Autodesk Fusion 360 part; units mm, degrees
note: some values were not read from the file. Set by a fixed rule: which face or edge a step refers to.
(part 2 of 2)
  spline S350 degree 3 poles (3.3037, -76.5729) (2.2719, -76.176) (1.5046, -77.2079) (2.1131, -78.1604) knots 0 0 0 0 1 1 1 1
  spline S351 degree 3 poles (2.1131, -78.1604) (2.4042, -78.6367) (4.9971, -78.769) (6.2142, -78.3456) knots 0 0 0 0 1 1 1 1
  spline S352 degree 3 poles (2.3248, -77.9488) (2.166, -77.79) (2.1131, -77.4725) (2.2189, -77.2344) knots 0 0 0 0 1 1 1 1
  spline S353 degree 3 poles (2.2189, -77.2344) (2.3512, -76.8904) (2.5894, -76.8375) (3.4889, -76.9698) knots 0 0 0 0 1 1 1 1
  spline S354 degree 3 poles (3.4889, -76.9698) (4.2298, -77.0756) (5.0235, -76.9963) (5.7908, -76.7052) knots 0 0 0 0 1 1 1 1
  spline S355 degree 3 poles (5.7908, -76.7052) (6.7962, -76.3613) (7.0344, -76.3613) (7.3254, -76.6523) knots 0 0 0 0 1 1 1 1
  spline S356 degree 3 poles (7.3254, -76.6523) (7.6164, -76.9433) (7.6164, -77.0756) (7.2196, -77.4196) knots 0 0 0 0 1 1 1 1
  spline S357 degree 3 poles (7.2196, -77.4196) (6.2142, -78.3456) (3.0392, -78.6631) (2.3248, -77.9488) knots 0 0 0 0 1 1 1 1
  spline S358 degree 3 poles (-4.3956, -78.425) (-3.0463, -78.1869) (-2.7552, -76.7052) (-3.9723, -76.3877) knots 0 0 0 0 1 1 1 1
  spline S359 degree 3 poles (-3.9723, -76.3877) (-4.475, -76.2554) (-4.475, -76.229) (-3.8929, -75.7263) knots 0 0 0 0 1 1 1 1
  line L74 (-3.8929, -75.7263) -> (-3.3108, -75.1971)
  line L75 (-3.3108, -75.1971) -> (-3.9723, -75.6204)
  spline S360 degree 3 poles (-3.9723, -75.6204) (-4.9248, -76.229) (-6.0096, -76.1496) (-6.7504, -75.3823) knots 0 0 0 0 1 1 1 1
  spline S361 degree 3 poles (-6.7504, -75.3823) (-7.5706, -74.5885) (-7.5971, -73.7154) (-6.8563, -72.71) knots 0 0 0 0 1 1 1 1
  line L76 (-6.8563, -72.71) -> (-6.3006, -71.9427)
  line L77 (-6.3006, -71.9427) -> (-6.9886, -72.6835)
  spline S362 degree 3 poles (-6.9886, -72.6835) (-7.359, -73.0804) (-7.6765, -73.7154) (-7.6765, -74.0858) knots 0 0 0 0 1 1 1 1
  spline S363 degree 3 poles (-7.6765, -74.0858) (-7.6765, -74.9854) (-6.3271, -76.3083) (-5.3746, -76.3348) knots 0 0 0 0 1 1 1 1
  spline S364 degree 3 poles (-5.3746, -76.3348) (-4.8983, -76.3613) (-4.7925, -76.4142) (-5.11, -76.4935) knots 0 0 0 0 1 1 1 1
  spline S365 degree 3 poles (-5.11, -76.4935) (-5.3746, -76.5729) (-6.1948, -76.4142) (-6.9356, -76.176) knots 0 0 0 0 1 1 1 1
  spline S366 degree 3 poles (-6.9356, -76.176) (-7.9411, -75.8585) (-8.3379, -75.8321) (-8.629, -76.0702) knots 0 0 0 0 1 1 1 1
  spline S367 degree 3 poles (-8.629, -76.0702) (-10.1106, -77.2873) (-7.1738, -78.9277) (-4.3956, -78.425) knots 0 0 0 0 1 1 1 1
  spline S368 degree 3 poles (-8.0204, -77.6313) (-9.4492, -76.9433) (-8.6819, -75.885) (-7.2002, -76.4935) knots 0 0 0 0 1 1 1 1
  spline S369 degree 3 poles (-7.2002, -76.4935) (-6.6711, -76.7052) (-5.7186, -76.8375) (-4.9248, -76.7846) knots 0 0 0 0 1 1 1 1
  spline S370 degree 3 poles (-4.9248, -76.7846) (-3.7871, -76.7052) (-3.5754, -76.7846) (-3.4961, -77.2079) knots 0 0 0 0 1 1 1 1
  spline S371 degree 3 poles (-3.4961, -77.2079) (-3.4431, -77.4725) (-3.549, -77.8165) (-3.7606, -77.9488) knots 0 0 0 0 1 1 1 1
  spline S372 degree 3 poles (-3.7606, -77.9488) (-4.2104, -78.2663) (-7.0944, -78.0546) (-8.0204, -77.6313) knots 0 0 0 0 1 1 1 1
  spline S373 degree 3 poles (-14.5027, -76.52) (-14.3175, -76.176) (-14.1588, -75.0119) (-14.1323, -73.7948) knots 0 0 0 0 1 1 1 1
  spline S374 degree 3 poles (-14.1323, -73.7948) (-14.1323, -72.419) (-13.9471, -71.3342) (-13.6825, -70.6992) knots 0 0 0 0 1 1 1 1
  spline S375 degree 3 poles (-13.6825, -70.6992) (-13.4444, -70.1435) (-13.2327, -69.6144) (-13.2327, -69.4821) knots 0 0 0 0 1 1 1 1
  spline S376 degree 3 poles (-13.2327, -69.4821) (-13.2327, -69.3498) (-13.0475, -69.0852) (-12.8358, -68.9) knots 0 0 0 0 1 1 1 1
  spline S377 degree 3 poles (-12.8358, -68.9) (-12.5448, -68.6619) (-12.2273, -68.6883) (-11.3013, -69.0323) knots 0 0 0 0 1 1 1 1
  spline S378 degree 3 poles (-11.3013, -69.0323) (-10.0842, -69.4821) (-5.745, -69.7202) (-4.475, -69.3763) knots 0 0 0 0 1 1 1 1
  spline S379 degree 3 poles (-4.475, -69.3763) (-3.9194, -69.2175) (-3.7342, -69.2969) (-3.4431, -69.826) knots 0 0 0 0 1 1 1 1
  spline S380 degree 3 poles (-3.4431, -69.826) (-3.0198, -70.5933) (-1.6704, -71.2813) (-0.5327, -71.2813) knots 0 0 0 0 1 1 1 1
  spline S381 degree 3 poles (-0.5327, -71.2813) (0.6314, -71.2813) (2.0602, -70.5404) (2.4835, -69.7467) knots 0 0 0 0 1 1 1 1
  spline S382 degree 3 poles (2.4835, -69.7467) (2.8275, -69.0588) (2.8275, -69.0588) (1.0019, -68.4502) knots 0 0 0 0 1 1 1 1
  spline S383 degree 3 poles (1.0019, -68.4502) (-0.2681, -68.0269) (-0.9561, -67.8946) (-1.1677, -68.0798) knots 0 0 0 0 1 1 1 1
  spline S384 degree 3 poles (-1.1677, -68.0798) (-1.3529, -68.2385) (-2.3319, -68.556) (-3.3373, -68.7942) knots 0 0 0 0 1 1 1 1
  spline S385 degree 3 poles (-3.3373, -68.7942) (-5.5069, -69.2969) (-9.555, -69.1646) (-11.3542, -68.5296) knots 0 0 0 0 1 1 1 1
  spline S386 degree 3 poles (-11.3542, -68.5296) (-12.9946, -67.921) (-13.1269, -67.974) (-13.4708, -69.244) knots 0 0 0 0 1 1 1 1
  spline S387 degree 3 poles (-13.4708, -69.244) (-13.6296, -69.879) (-13.9736, -70.6992) (-14.2646, -71.0431) knots 0 0 0 0 1 1 1 1
  spline S388 degree 3 poles (-14.2646, -71.0431) (-14.7144, -71.6252) (-14.7408, -71.8633) (-14.5027, -73.0804) knots 0 0 0 0 1 1 1 1
  spline S389 degree 3 poles (-14.5027, -73.0804) (-14.2911, -74.1652) (-14.3175, -74.6944) (-14.635, -75.6998) knots 0 0 0 0 1 1 1 1
  spline S390 degree 3 poles (-14.635, -75.6998) (-15.1113, -77.1021) (-15.0319, -77.4725) (-14.5027, -76.52) knots 0 0 0 0 1 1 1 1
  line L78 (-2.8611, -70.0642) -> (-3.4696, -69.3498)
  line L79 (-3.4696, -69.3498) -> (-2.0938, -68.9)
  spline S391 degree 3 poles (-2.0938, -68.9) (-0.5063, -68.3444) (-0.4004, -68.3444) (0.7373, -69.0323) knots 0 0 0 0 1 1 1 1
  spline S392 degree 3 poles (0.7373, -69.0323) (1.7692, -69.6408) (1.7162, -69.9319) (0.4992, -70.5669) knots 0 0 0 0 1 1 1 1
  spline S393 degree 3 poles (0.4992, -70.5669) (-0.6915, -71.2019) (-2.0673, -70.9902) (-2.8611, -70.0642) knots 0 0 0 0 1 1 1 1
  spline S394 degree 3 poles (2.0337, -69.5615) (2.1131, -69.3233) (2.2454, -69.191) (2.2983, -69.2704) knots 0 0 0 0 1 1 1 1
  spline S395 degree 3 poles (2.2983, -69.2704) (2.3777, -69.3498) (2.3512, -69.5085) (2.2454, -69.6673) knots 0 0 0 0 1 1 1 1
  spline S396 degree 3 poles (2.2454, -69.6673) (2.0073, -70.0906) (1.8485, -70.0113) (2.0337, -69.5615) knots 0 0 0 0 1 1 1 1
  spline S397 degree 3 poles (-0.2681, -70.514) (-0.2681, -70.3817) (0.0229, -70.1965) (0.3933, -70.1171) knots 0 0 0 0 1 1 1 1
  spline S398 degree 3 poles (0.3933, -70.1171) (0.7637, -70.0113) (1.0548, -69.826) (1.0548, -69.6938) knots 0 0 0 0 1 1 1 1
  spline S399 degree 3 poles (1.0548, -69.6938) (1.0548, -69.5615) (0.7373, -69.5615) (0.261, -69.7202) knots 0 0 0 0 1 1 1 1
  spline S400 degree 3 poles (0.261, -69.7202) (-0.1888, -69.879) (-0.5327, -70.17) (-0.5327, -70.3817) knots 0 0 0 0 1 1 1 1
  spline S401 degree 3 poles (-0.5327, -70.3817) (-0.5327, -70.5933) (-0.4798, -70.7521) (-0.4004, -70.7521) knots 0 0 0 0 1 1 1 1
  spline S402 degree 3 poles (-0.4004, -70.7521) (-0.3211, -70.7521) (-0.2681, -70.6463) (-0.2681, -70.514) knots 0 0 0 0 1 1 1 1
  spline S403 degree 3 poles (4.0446, -76.0438) (3.5683, -75.9379) (3.0127, -75.7527) (2.8275, -75.6204) knots 0 0 0 0 1 1 1 1
  spline S404 degree 3 poles (2.8275, -75.6204) (2.6423, -75.4881) (2.7217, -75.594) (2.9862, -75.8585) knots 0 0 0 0 1 1 1 1
  spline S405 degree 3 poles (2.9862, -75.8585) (3.2773, -76.0967) (3.8064, -76.3083) (4.2033, -76.2819) knots 0 0 0 0 1 1 1 1
  spline S406 degree 3 poles (4.2033, -76.2819) (4.8383, -76.2554) (4.8119, -76.229) (4.0446, -76.0438) knots 0 0 0 0 1 1 1 1
  spline S407 degree 3 poles (5.8967, -75.5675) (6.1612, -75.3029) (6.3464, -74.8531) (6.32, -74.5621) knots 0 0 0 0 1 1 1 1
  spline S408 degree 3 poles (6.32, -74.5621) (6.32, -74.1917) (6.2671, -74.1652) (6.1612, -74.4563) knots 0 0 0 0 1 1 1 1
  spline S409 degree 3 poles (6.1612, -74.4563) (6.0819, -74.6679) (5.7644, -75.1177) (5.4733, -75.4617) knots 0 0 0 0 1 1 1 1
  spline S410 degree 3 poles (5.4733, -75.4617) (5.1823, -75.7792) (5.05, -76.0438) (5.2087, -76.0438) knots 0 0 0 0 1 1 1 1
  spline S411 degree 3 poles (5.2087, -76.0438) (5.341, -76.0438) (5.6585, -75.8321) (5.8967, -75.5675) knots 0 0 0 0 1 1 1 1
  spline S412 degree 3 poles (-3.9458, -74.6944) (-3.2315, -73.98) (-3.3638, -72.8688) (-4.2633, -72.366) knots 0 0 0 0 1 1 1 1
  spline S413 degree 3 poles (-4.2633, -72.366) (-4.8983, -72.0221) (-5.0306, -72.0221) (-5.6656, -72.419) knots 0 0 0 0 1 1 1 1
  spline S414 degree 3 poles (-5.6656, -72.419) (-6.38, -72.8952) (-6.6446, -74.2446) (-6.089, -74.5885) knots 0 0 0 0 1 1 1 1
  spline S415 degree 3 poles (-6.089, -74.5885) (-5.9567, -74.6679) (-5.8244, -74.615) (-5.8244, -74.4827) knots 0 0 0 0 1 1 1 1
  spline S416 degree 3 poles (-5.8244, -74.4827) (-5.8244, -74.324) (-5.6392, -74.1917) (-5.4011, -74.1917) knots 0 0 0 0 1 1 1 1
  spline S417 degree 3 poles (-5.4011, -74.1917) (-5.11, -74.1917) (-5.0042, -74.3504) (-5.11, -74.7208) knots 0 0 0 0 1 1 1 1
  spline S418 degree 3 poles (-5.11, -74.7208) (-5.2952, -75.4352) (-4.6602, -75.4088) (-3.9458, -74.6944) knots 0 0 0 0 1 1 1 1
  spline S419 degree 3 poles (-5.3746, -73.2392) (-5.3481, -73.1069) (-5.0836, -72.9746) (-4.819, -72.9217) knots 0 0 0 0 1 1 1 1
  spline S420 degree 3 poles (-4.819, -72.9217) (-4.2898, -72.8423) (-3.84, -73.5038) (-4.1311, -73.9535) knots 0 0 0 0 1 1 1 1
  spline S421 degree 3 poles (-4.1311, -73.9535) (-4.3163, -74.271) (-5.454, -73.5831) (-5.3746, -73.2392) knots 0 0 0 0 1 1 1 1
  spline S422 degree 3 poles (3.8594, -74.7473) (3.78, -74.615) (3.8858, -74.3769) (4.071, -74.2181) knots 0 0 0 0 1 1 1 1
  spline S423 degree 3 poles (4.071, -74.2181) (4.3621, -73.9535) (4.5208, -74.0065) (4.706, -74.3769) knots 0 0 0 0 1 1 1 1
  spline S424 degree 3 poles (4.706, -74.3769) (4.9442, -74.8002) (4.9971, -74.7473) (5.1823, -74.0858) knots 0 0 0 0 1 1 1 1
  spline S425 degree 3 poles (5.1823, -74.0858) (5.4998, -72.7629) (4.4944, -71.784) (3.2508, -72.2338) knots 0 0 0 0 1 1 1 1
  spline S426 degree 3 poles (3.2508, -72.2338) (1.9544, -72.6835) (2.1396, -74.9854) (3.4889, -74.9854) knots 0 0 0 0 1 1 1 1
  spline S427 degree 3 poles (3.4889, -74.9854) (3.7535, -74.9854) (3.9387, -74.8796) (3.8594, -74.7473) knots 0 0 0 0 1 1 1 1
  spline S428 degree 3 poles (3.0921, -73.4508) (3.3302, -72.8158) (3.7535, -72.5777) (4.1504, -72.9217) knots 0 0 0 0 1 1 1 1
  spline S429 degree 3 poles (4.1504, -72.9217) (4.415, -73.1333) (4.3621, -73.2921) (3.8858, -73.6625) knots 0 0 0 0 1 1 1 1
  spline S430 degree 3 poles (3.8858, -73.6625) (3.2244, -74.2181) (2.8539, -74.1123) (3.0921, -73.4508) knots 0 0 0 0 1 1 1 1
  spline S431 degree 3 poles (6.32, -73.3715) (6.3464, -73.1333) (6.0819, -72.7365) (5.7379, -72.4454) knots 0 0 0 0 1 1 1 1
  spline S432 degree 3 poles (5.7379, -72.4454) (5.1558, -71.9427) (5.1558, -71.9427) (5.5792, -72.4719) knots 0 0 0 0 1 1 1 1
  spline S433 degree 3 poles (5.5792, -72.4719) (5.8173, -72.7629) (6.0819, -73.1863) (6.1612, -73.3979) knots 0 0 0 0 1 1 1 1
  spline S434 degree 3 poles (6.1612, -73.3979) (6.2935, -73.7419) (6.32, -73.7419) (6.32, -73.3715) knots 0 0 0 0 1 1 1 1
  spline S435 degree 3 poles (13.2256, -65.3017) (13.2256, -63.4231) (7.881, -61.5446) (4.3092, -62.1796) knots 0 0 0 0 1 1 1 1
  spline S436 degree 3 poles (4.3092, -62.1796) (3.145, -62.3913) (3.2773, -62.4177) (5.9496, -62.5765) knots 0 0 0 0 1 1 1 1
  spline S437 degree 3 poles (5.9496, -62.5765) (7.5371, -62.6823) (9.2833, -62.894) (9.8125, -63.0527) knots 0 0 0 0 1 1 1 1
  spline S438 degree 3 poles (9.8125, -63.0527) (11.1089, -63.4496) (12.4848, -64.4021) (12.8817, -65.1958) knots 0 0 0 0 1 1 1 1
  spline S439 degree 3 poles (12.8817, -65.1958) (13.1992, -65.8308) (13.2256, -65.8308) (13.2256, -65.3017) knots 0 0 0 0 1 1 1 1
  spline S440 degree 3 poles (-13.8148, -64.6667) (-13.0475, -63.4231) (-10.0577, -62.55) (-6.5388, -62.55) knots 0 0 0 0 1 1 1 1
  spline S441 degree 3 poles (-6.5388, -62.55) (-4.819, -62.5235) (-4.475, -62.4706) (-4.8719, -62.2325) knots 0 0 0 0 1 1 1 1
  spline S442 degree 3 poles (-4.8719, -62.2325) (-5.5333, -61.8621) (-9.1846, -62.1267) (-11.0896, -62.7088) knots 0 0 0 0 1 1 1 1
  spline S443 degree 3 poles (-11.0896, -62.7088) (-12.3861, -63.0792) (-14.6086, -64.6931) (-14.2911, -65.0371) knots 0 0 0 0 1 1 1 1
  spline S444 degree 3 poles (-14.2911, -65.0371) (-14.2117, -65.1165) (-14, -64.9313) (-13.8148, -64.6667) knots 0 0 0 0 1 1 1 1
  spline S445 degree 3 poles (0.2081, -63.529) (0.7637, -63.2115) (0.6844, -63.185) (-0.5327, -63.185) knots 0 0 0 0 1 1 1 1
  spline S446 degree 3 poles (-0.5327, -63.185) (-1.7498, -63.185) (-1.8292, -63.2115) (-1.2736, -63.529) knots 0 0 0 0 1 1 1 1
  spline S447 degree 3 poles (-1.2736, -63.529) (-0.9296, -63.7142) (-0.6121, -63.8465) (-0.5327, -63.8465) knots 0 0 0 0 1 1 1 1
  spline S448 degree 3 poles (-0.5327, -63.8465) (-0.4533, -63.8465) (-0.1358, -63.7142) (0.2081, -63.529) knots 0 0 0 0 1 1 1 1
  spline S449 degree 3 poles (2.6158, -62.3648) (1.3458, -60.8567) (-2.7023, -60.8831) (-3.9988, -62.4442) knots 0 0 0 0 1 1 1 1
  spline S450 degree 3 poles (-3.9988, -62.4442) (-4.2633, -62.7617) (-3.7606, -62.8146) (-0.665, -62.8146) knots 0 0 0 0 1 1 1 1
  spline S451 degree 3 poles (-0.665, -62.8146) (2.6952, -62.8146) (2.9333, -62.7881) (2.6158, -62.3648) knots 0 0 0 0 1 1 1 1
  spline S452 degree 3 poles (-0.6121, -61.8356) (-0.4269, -61.7827) (-0.1094, -61.7827) (0.0494, -61.8356) knots 0 0 0 0 1 1 1 1
  spline S453 degree 3 poles (0.0494, -61.8356) (0.2346, -61.915) (0.1023, -61.9679) (-0.2681, -61.9679) knots 0 0 0 0 1 1 1 1
  spline S454 degree 3 poles (-0.2681, -61.9679) (-0.6386, -61.9679) (-0.7708, -61.915) (-0.6121, -61.8356) knots 0 0 0 0 1 1 1 1
  spline S455 degree 3 poles (0.896, -33.4723) (1.0812, -33.1813) (-0.1358, -32.9431) (-0.5327, -33.1813) knots 0 0 0 0 1 1 1 1
  spline S456 degree 3 poles (-0.5327, -33.1813) (-0.7444, -33.3135) (-0.6915, -33.4194) (-0.4004, -33.5517) knots 0 0 0 0 1 1 1 1
  spline S457 degree 3 poles (-0.4004, -33.5517) (0.2081, -33.7898) (0.7373, -33.7633) (0.896, -33.4723) knots 0 0 0 0 1 1 1 1
  spline S458 degree 3 poles (3.0656, -30.7206) (3.145, -30.509) (3.1714, -29.4242) (3.1185, -28.26) knots 0 0 0 0 1 1 1 1
  line L80 (3.1185, -28.26) -> (3.0392, -26.1698)
  line L81 (3.0392, -26.1698) -> (0.261, -26.1698)
  line L82 (0.261, -26.1698) -> (-2.5171, -26.1698)
  line L83 (-2.5171, -26.1698) -> (-2.5171, -28.551)
  line L84 (-2.5171, -28.551) -> (-2.5171, -30.9323)
  line L85 (-2.5171, -30.9323) -> (0.2081, -31.0117)
  spline S459 degree 3 poles (0.2081, -31.0117) (2.3248, -31.0646) (2.9598, -31.0117) (3.0656, -30.7206) knots 0 0 0 0 1 1 1 1
  spline S460 degree 3 poles (-1.9615, -30.6413) (-2.3054, -30.509) (-2.3848, -30.0592) (-2.3848, -28.5246) knots 0 0 0 0 1 1 1 1
  line L86 (-2.3848, -28.5246) -> (-2.3848, -26.5667)
  line L87 (-2.3848, -26.5667) -> (0.2346, -26.5667)
  line L88 (0.2346, -26.5667) -> (2.8275, -26.5667)
  line L89 (2.8275, -26.5667) -> (2.8804, -28.4188)
  spline S461 degree 3 poles (2.8804, -28.4188) (2.9069, -29.4506) (2.8539, -30.4031) (2.7746, -30.5354) knots 0 0 0 0 1 1 1 1
  spline S462 degree 3 poles (2.7746, -30.5354) (2.5894, -30.8265) (-1.2736, -30.9058) (-1.9615, -30.6413) knots 0 0 0 0 1 1 1 1
  spline S463 degree 3 poles (0.9754, -23.8679) (0.9225, -23.6827) (0.5521, -23.524) (0.1287, -23.524) knots 0 0 0 0 1 1 1 1
  spline S464 degree 3 poles (0.1287, -23.524) (-0.2946, -23.524) (-0.665, -23.6827) (-0.7444, -23.8679) knots 0 0 0 0 1 1 1 1
  spline S465 degree 3 poles (-0.7444, -23.8679) (-0.7973, -24.0796) (-0.5327, -24.1854) (0.1287, -24.1854) knots 0 0 0 0 1 1 1 1
  spline S466 degree 3 poles (0.1287, -24.1854) (0.7902, -24.1854) (1.0548, -24.0796) (0.9754, -23.8679) knots 0 0 0 0 1 1 1 1
  spline S467 degree 3 poles (-26.6206, -72.8688) (-24.6627, -71.6252) (-23.525, -68.556) (-24.3452, -66.651) knots 0 0 0 0 1 1 1 1
  spline S468 degree 3 poles (-24.3452, -66.651) (-24.4775, -66.3071) (-24.504, -66.6246) (-24.4246, -67.4713) knots 0 0 0 0 1 1 1 1
  spline S469 degree 3 poles (-24.4246, -67.4713) (-24.16, -69.9054) (-25.4565, -72.1808) (-27.6525, -73.1598) knots 0 0 0 0 1 1 1 1
  spline S470 degree 3 poles (-27.6525, -73.1598) (-28.2346, -73.4244) (-28.5256, -73.6625) (-28.2875, -73.6625) knots 0 0 0 0 1 1 1 1
  spline S471 degree 3 poles (-28.2875, -73.6625) (-28.0758, -73.6625) (-27.335, -73.2921) (-26.6206, -72.8688) knots 0 0 0 0 1 1 1 1
  spline S472 degree 3 poles (-12.7829, -32.2023) (-12.439, -32.1494) (-12.1744, -31.9906) (-12.1744, -31.8583) knots 0 0 0 0 1 1 1 1
  spline S473 degree 3 poles (-12.1744, -31.8583) (-12.1744, -31.726) (-12.5448, -31.726) (-12.9946, -31.8583) knots 0 0 0 0 1 1 1 1
  spline S474 degree 3 poles (-12.9946, -31.8583) (-14.4498, -32.2817) (-14.3175, -32.4933) (-12.7829, -32.2023) knots 0 0 0 0 1 1 1 1
  spline S475 degree 3 poles (-9.6608, -31.5673) (-9.0788, -31.4615) (-8.1263, -31.3556) (-7.5706, -31.3556) knots 0 0 0 0 1 1 1 1
  spline S476 degree 3 poles (-7.5706, -31.3556) (-6.8827, -31.3292) (-6.5917, -31.2498) (-6.7769, -31.0646) knots 0 0 0 0 1 1 1 1
  spline S477 degree 3 poles (-6.7769, -31.0646) (-7.015, -30.8265) (-11.5658, -31.435) (-11.8833, -31.7525) knots 0 0 0 0 1 1 1 1
  spline S478 degree 3 poles (-11.8833, -31.7525) (-12.0686, -31.9113) (-10.8515, -31.8319) (-9.6608, -31.5673) knots 0 0 0 0 1 1 1 1
  spline S479 degree 3 poles (16.0567, -32.6521) (15.5804, -32.361) (15.0777, -32.2023) (13.6225, -31.9642) knots 0 0 0 0 1 1 1 1
  spline S480 degree 3 poles (13.6225, -31.9642) (13.1727, -31.8848) (12.3525, -31.6996) (11.7704, -31.5673) knots 0 0 0 0 1 1 1 1
  spline S481 degree 3 poles (11.7704, -31.5673) (10.2358, -31.1969) (9.5214, -31.1175) (9.5214, -31.3027) knots 0 0 0 0 1 1 1 1
  spline S482 degree 3 poles (9.5214, -31.3027) (9.5214, -31.3821) (10.8708, -31.726) (12.5112, -32.0435) knots 0 0 0 0 1 1 1 1
  spline S483 degree 3 poles (12.5112, -32.0435) (14.1517, -32.361) (15.7127, -32.705) (16.0037, -32.7844) knots 0 0 0 0 1 1 1 1
  spline S484 degree 3 poles (16.0037, -32.7844) (16.48, -32.9431) (16.48, -32.9431) (16.0567, -32.6521) knots 0 0 0 0 1 1 1 1
  spline S485 degree 3 poles (-25.9592, -25.1115) (-25.0331, -24.8998) (-24.2394, -24.6881) (-24.1865, -24.6352) knots 0 0 0 0 1 1 1 1
  spline S486 degree 3 poles (-24.1865, -24.6352) (-24.1336, -24.5823) (-24.16, -23.7885) (-24.2658, -22.8625) knots 0 0 0 0 1 1 1 1
  spline S487 degree 3 poles (-24.2658, -22.8625) (-24.4246, -21.1427) (-25.0861, -20.0315) (-25.8004, -20.3225) knots 0 0 0 0 1 1 1 1
  spline S488 degree 3 poles (-25.8004, -20.3225) (-26.0386, -20.4019) (-26.1973, -20.0844) (-26.3296, -19.2377) knots 0 0 0 0 1 1 1 1
  spline S489 degree 3 poles (-26.3296, -19.2377) (-26.4354, -18.4704) (-26.7529, -17.7825) (-27.1763, -17.3592) knots 0 0 0 0 1 1 1 1
  spline S490 degree 3 poles (-27.1763, -17.3592) (-27.8113, -16.7242) (-27.9171, -16.7242) (-29.9808, -16.8829) knots 0 0 0 0 1 1 1 1
  spline S491 degree 3 poles (-29.9808, -16.8829) (-33.7115, -17.2004) (-34.1083, -17.7825) (-33.6321, -22.1746) knots 0 0 0 0 1 1 1 1
  line L90 (-33.6321, -22.1746) -> (-33.2881, -25.1644)
  line L91 (-33.2881, -25.1644) -> (-31.6742, -25.3496)
  spline S492 degree 3 poles (-31.6742, -25.3496) (-29.3988, -25.5877) (-27.8906, -25.5083) (-25.9592, -25.1115) knots 0 0 0 0 1 1 1 1
  line L92 (-31.8594, -24.5558) -> (-33.0765, -24.3706)
  line L93 (-33.0765, -24.3706) -> (-33.1029, -23.1535)
  spline S493 degree 3 poles (-33.1029, -23.1535) (-33.1029, -22.4921) (-33.2088, -21.3808) (-33.3146, -20.6929) knots 0 0 0 0 1 1 1 1
  spline S494 degree 3 poles (-33.3146, -20.6929) (-33.5527, -19.1583) (-33.1029, -17.9148) (-32.2298, -17.7031) knots 0 0 0 0 1 1 1 1
  spline S495 degree 3 poles (-32.2298, -17.7031) (-30.6952, -17.3592) (-28.3404, -17.174) (-27.8906, -17.3592) knots 0 0 0 0 1 1 1 1
  spline S496 degree 3 poles (-27.8906, -17.3592) (-27.335, -17.6238) (-26.7265, -18.735) (-26.7265, -19.5023) knots 0 0 0 0 1 1 1 1
  spline S497 degree 3 poles (-26.7265, -19.5023) (-26.7265, -20.2431) (-26.2238, -21.0104) (-25.8269, -20.8517) knots 0 0 0 0 1 1 1 1
  spline S498 degree 3 poles (-25.8269, -20.8517) (-25.2977, -20.64) (-24.9273, -21.3015) (-24.8215, -22.7302) knots 0 0 0 0 1 1 1 1
  line L94 (-24.8215, -22.7302) -> (-24.7421, -24.0531)
  line L95 (-24.7421, -24.0531) -> (-26.1973, -24.3706)
  spline S499 degree 3 poles (-26.1973, -24.3706) (-27.8906, -24.7146) (-30.0867, -24.794) (-31.8594, -24.5558) knots 0 0 0 0 1 1 1 1
  line L96 (20.8721, -39.0021) -> (21.3748, -39.399)
  line L97 (-33.9761, -24.9792) -> (-33.2881, -25.1644)
  line L98 (-24.1865, -24.6352) -> (-22.89, -24.45)
  line L99 (-20.4346, -3.0717) -> (-20.1383, -2.3838)
  line L100 (3.3831, -3.2833) -> (4.5234, -3.872)
  constraint coincident S111 L99.start
  constraint coincident S86 L100.end
sketch "Schizzo2" plane through (0, 0, 0) normal (0, 0, 1) x (1, 0, 0)
  circle A0 centre (0, 0) radius 43
  constraint coincident A0.centre origin
extrude "Estrudi1" add sketch "Schizzo2" along normal blind 106 makes body 1
shell "Shell1" thickness 3 removed faces 1 at (3.1895, 5.5243, 106) on bodies 1
extrude "Estrudi2" add sketch "Schizzo1" along normal up to surface separate body contours S0 S1 S2 L0 L1 S3 S4 S5 S6 S7 S8 S9 S10 S11 S12 S13 S14 S15 S16 S17 S18 S19 S20 S21 S22 S23 S24 S25 S26 S27 S28 S29 S30 S31 S32 S33 S34 S35 S36 S37 S38 S39 S40 S41 S42 S43 S44 S45 S46 S47 S48 S49 S50 S51 S52 S53 S54 S55 L2 L3 L4 L5 S56 L6 L7 L8 L9 L10 L11 S57 S58 S59 S60 S61 S62 S63 S64 S65 S66 S67 S68 S69 S70 S71 S72 S73 S74 S75 S76 S77 S78 S79 S80 S81 S82 S83 S84 S85 L12 L13 S86 L14 L15 S87 S88 S89 S90 S91 S92 S93 L16 L17 L18 L19 S94 L20 L21 S95 S96 S97 S98 S99 S100 S101 L22 L23 S102 S103 S104 L24 L25 S105 S106 S107 S108 S109 S110 S111 S112 S113 S114 L26 L27 S115 S116 S117 S118 S119 S120 S121 S122 S123 S124 S125 S126 S127 S128 S129 S130 S131 S132 S133 S134 S135 S136 L28 L29 S137 S138 S139 S140 S141 S142 S143 S144 S145 S146 S147 S148 S149 L96 L97 L100 | S27 S28 S29 S30 S31 S32 S33 S34 S35 S36 S37 S38 S39 S40 S41 S42 S43 S44 S45 S46 S47 S48 S49 S50 S51 S52 S53 S54 S55 L2 L3 L4 L5 S56 L6 L7 L8 L9 L10 L11 S57 S58 S59 S60 S61 S62 S63 S64 S65 S66 S67 S68 S69 S70 S71 S72 L96 | S150 S151 S152 S153 S154 S155 S156 L30 L31 S157 S158 S159 S160 S161 L32 L33 S162 S163 S164 S165 S166 S167 S168 S169 S170 S171 S172 S173 S174 S175 S176 S177 | S303 S304 S305 S306 S307 S308 S309 | S310 S311 S312 L72 L73 S313 S314 | S315 S316 S317 S318 S319 S320 | S352 S353 S354 S355 S356 S357 | S368 S369 S370 S371 S372 | L78 L79 S391 S392 S393 | S445 S446 S447 S448 | L92 L93 S493 S494 S495 S496 S497 S498 L94 L95 S499 end surface at (42.9465, -2.1434, 70.6667) on bodies 1 makes body 2 at (0.0965, -19.1101, 70.7474) makes body 3 at (-16.5536, -39.686, 22.5443) makes body 4 at (-0.1685, -19.11, 63.1863) makes body 5 at (4.4953, -8.3489, 78.3151) makes body 6 at (-6.31, -35.4994, 78.0104) makes body 7 at (-30.0233, -27.4365, 24.6893)
move_body "Sposta1" bodies 6 3 4 5 7 2 to x (1, 0, 0) y (0, 1, 0) z (0, 0, 1) at (0, -5, 0)
sketch "Schizzo3" plane through (0, 0, 0) normal (0, 0, 1) x (1, 0, 0)
  circle A0 centre (0, 0) radius 40.1123
  constraint coincident A0.centre origin
extrude "Estrudi3" cut 1 faces at (-17.1478, 1.6902, 3) along direction (0, 0, 1) blind 138 on bodies 1 bodies 2 3 4 5 6 7
combine "Unisci1" operation add target body 7 tool bodies 1 5 2 4 6 3
